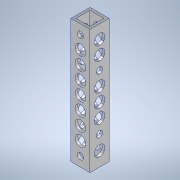
# Autodesk Inventor part: 上下直動9x9_4
Saved by Autodesk Inventor 2020.3 (Build 243373000, 373)
## iProperties
Created: 2020-07-07
Part Number: 上下直動9x9_4
Material: アルミニウム 6061
Document SubType Name: Modeling
Designer: totot
Density: 2.7 g/cm^3
Appearance: アルミニウム - フラット
Mass: 5.73043 g
Surface Area: 37.0266 cm^2
Volume: 2.12238 cm^3
Author: totot
Autodesk Inventor part; units mm, degrees
ref_plane "YZ Plane" through (0, 0, 0) normal (1, 0, 0) x (0, 1, 0)
ref_plane "XZ Plane" through (0, 0, 0) normal (0, 1, 0) x (-1, 0, 0)
ref_plane "XY Plane" through (0, 0, 0) normal (0, 0, 1) x (1, 0, 0)
sketch "スケッチ1" plane through (0, 0, 0) normal (0, 1, 0) x (-1, 0, 0)
  line L0 (0, 0) -> (-9, 0)
  line L1 (-9, 0) -> (-9, 9)
  line L2 (-9, 9) -> (0, 9)
  line L3 (0, 9) -> (0, 0)
  line L4 (-1.2, 7.8) -> (-7.8, 7.8)
  line L5 (-7.8, 7.8) -> (-7.8, 1.2)
  line L6 (-7.8, 1.2) -> (-1.2, 1.2)
  line L7 (-1.2, 1.2) -> (-1.2, 7.8)
  dimension "d0" = 9
  dimension "d1" = 9
  dimension "d2" = 6.6
  dimension "d3" = 6.6
  dimension "d4" = 1.2
  dimension "d5" = 1.2
  constraints: 16 end point, 4 parallel, 2 horizontal, 2 perpendicular
  measures "d0" distance of L1.end L2.end
  measures "d1" distance of L0.end L1.end
  measures "d2" distance of L6.end L5.end
  measures "d3" distance of L5.end L4.end
  measures "d4" distance between parallel lines of L7 L3
  measures "d5" distance between parallel lines of L4 L2
extrude "押し出し1" add sketch "スケッチ1" along normal blind 58.5
sketch "スケッチ2" plane through (0, 0, 9) normal (0, 0, 1) x (1, 0, 0)
  line L0 (0, 58.5) -> (9, 58.5) projected
  line L1 (9, 0) -> (9, 58.5) projected
  line L2 (0, 0) -> (9, 0) projected
  point P0 (4.5, 4.5)
  point P1 (4.5, 54)
  dimension "d8" = 4.5
  dimension "d9" = 4.5
  dimension "d10" = 4.5
  dimension "d11" = 4.5
  measures "d8" distance from line of point (4.5, 54) L0
  measures "d9" distance from line of point (4.5, 54) L1
  measures "d10" distance from line of L1 point (4.5, 4.5)
  measures "d11" distance from line of point (4.5, 4.5) L2
hole "穴1" at (4.5, 4.5, 9) at (4.5, 54, 9) direction (0, 0, -1) diameter 3 end through all
sketch "スケッチ3" plane through (9, 0, 9) normal (1, 0, 0) x (0, 0, -1)
  line L0 (0, 0) -> (9, 0) projected
  line L1 (0, 0) -> (0, 58.5) projected
  line L2 (0, 58.5) -> (9, 58.5) projected
  point P0 (4.5, 13.5)
  point P1 (4.5, 39.5)
  dimension "d19" = 13.5
  dimension "d20" = 4.5
  dimension "d21" = 19
  dimension "d22" = 4.5
  measures "d19" distance from line of L0 point (4.5, 13.5)
  measures "d20" distance from line of L1 point (4.5, 13.5)
  measures "d21" distance from line of point (4.5, 39.5) L2
  measures "d22" distance from line of point (4.5, 39.5) L1
hole "穴2" at (9, 13.5, 4.5) at (9, 39.5, 4.5) direction (-1, 0, 0) diameter 3 end through all
sketch "スケッチ4" plane through (0, 0, 0) normal (-1, 0, 0) x (0, 0, 1)
  line L0 (9, 0) -> (0, 0) projected
  line L1 (4.5, 0) -> (4.5, 58.5)
  line L2 (1.2, 58.5) -> (7.8, 58.5) projected
  line L3 (0, 0) -> (0, 58.5) projected
  circle A0 centre (4.5, 13.5) radius 1.5 projected
  circle A1 centre (4.5, 39.5) radius 1.5 projected
  point P0 (4.5, 6.75)
  point P1 (4.5, 20)
  point P2 (4.5, 33)
  point P3 (4.5, 45.8333)
  point P4 (4.5, 52.1667)
  point P5 (4.5, 26.5)
  dimension "d30" = 4.5
  dimension "d31" = 13.5
  dimension "d32" = 6.75
  dimension "d33" = 26
  dimension "d34" = 6.5
  dimension "d35" = 6.5
  dimension "d36" = 6.5
  dimension "d37" = 19
  dimension "d38" = 6.3333
  dimension "d39" = 6.3333
  constraints: 6 point on line, 2 end point, 2 midpoint
  measures "d30" distance between parallel lines of L1 L3
  measures "d31" distance from line of A0.centre L0
  measures "d32" distance of A0.centre point (4.5, 6.75)
  measures "d33" distance of A1.centre A0.centre
  measures "d34" distance of point (4.5, 20) A0.centre
  measures "d35" distance of point (4.5, 26.5) point (4.5, 20)
  measures "d36" distance of point (4.5, 26.5) point (4.5, 33)
  measures "d37" distance from line of L2 A1.centre
  measures "d38" distance of point (4.5, 45.833) A1.centre
  measures "d39" distance of point (4.5, 45.833) point (4.5, 52.167)
hole "穴3" at (0, 6.75, 4.5) at (0, 20, 4.5) at (0, 33, 4.5) at (0, 45.8333, 4.5) at (0, 52.1667, 4.5) at (0, 26.5, 4.5) direction (1, 0, 0) diameter 5 end through all
sketch "スケッチ5" plane through (9, 0, 0) normal (0, 0, -1) x (-1, 0, 0)
  circle A0 centre (4.5, 4.5) radius 1.5 projected
  circle A1 centre (4.5, 54) radius 1.5 projected
  line L0 (4.5, 4.5) -> (4.5, 54)
  point P0 (9, 0)
  point P1 (4.5, 10.6875)
  point P2 (4.5, 16.875)
  point P3 (4.5, 23.0625)
  point P4 (4.5, 29.25)
  point P5 (4.5, 35.4375)
  point P6 (4.5, 41.625)
  point P7 (4.5, 47.8125)
  dimension "d47" = 49.5
  dimension "d48" = 6.1875
  dimension "d51" = 6.1875
  constraints: 2 end point, 2 vertical, 1 point on line, 6 other
  measures "d47" distance of L0.start L0.end
  measures "d48" distance of point (4.5, 10.687) L0.start
  measures "d51" distance of point (4.5, 10.687) point (4.5, 16.875)
hole "穴4" at (4.5, 10.6875, 0) at (4.5, 16.875, 0) at (4.5, 23.0625, 0) at (4.5, 29.25, 0) at (4.5, 35.4375, 0) at (4.5, 41.625, 0) at (4.5, 47.8125, 0) direction (0, 0, 1) diameter 5 end through all
equation "\"d5\" = d4"
equation "\"d9\" = d8"
equation "\"d11\" = d10"
equation "\"d32\" = 0.5 * d31"
equation "\"d34\" = 0.25 * d33"
equation "\"d35\" = d34"
equation "\"d36\" = d35"
equation "\"d38\" = 0.333333 * d37"
equation "\"d39\" = d38"
equation "\"d48\" = 0.125 * d47"
